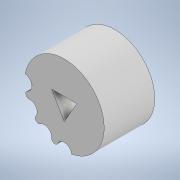
# Autodesk Inventor part: HandleGear
Saved by Autodesk Inventor 2021 (Build 250183000, 183)
## iProperties
Created: 2021-03-14
Part Number: HandleGear
Material: Generic
Document SubType Name: Modeling
Designer: ben
Density: 1 g/cm^3
Appearance: Default
Author: ben
Autodesk Inventor part; units mm, degrees
ref_plane "YZ Plane" through (0, 0, 0) normal (1, 0, 0) x (0, 1, 0)
ref_plane "XZ Plane" through (0, 0, 0) normal (0, 1, 0) x (-1, 0, 0)
ref_plane "XY Plane" through (0, 0, 0) normal (0, 0, 1) x (1, 0, 0)
sketch "Sketch1" plane through (0, 0, 0) normal (0, 0, 1) x (1, 0, 0)
  line L0 (4.323, -2.5122) -> (-0.0282, -10) projected
  line L1 (-0.0282, -10) -> (-4.3372, -2.4878) projected
  line L2 (-8.6461, 5.0244) -> (0.0141, 5) projected
  circle A0 centre (0, 0) radius 27.5 projected
  circle A1 centre (0, 0) radius 22.5
  line L3 (0, 27.5) -> (0, 14.4902)
  line L4 (0, 0) -> (27.5, 0) construction
  line L5 (0, 0) -> (27.5, 0) construction
  circle A2 centre (-27.5, 0) radius 5
  circle A3 centre (-23.8157, -13.75) radius 5
  circle A4 centre (-13.75, -23.8157) radius 5
  circle A5 centre (0, -27.5) radius 5
  line L6 (-4.3372, -2.4878) -> (-8.6461, 5.0244) projected
  line L7 (0.0141, 5) -> (8.6743, 4.9755) projected
  line L8 (8.6743, 4.9755) -> (4.323, -2.5122) projected
  point P0 (0, 0)
  point P1 (-27.0822, 4.7753)
  point P2 (4.7753, -27.0822)
  point P3 (-4.9793, -27.0455)
  point P4 (4.9793, -27.0455)
  point P5 (-27.0455, 4.9793)
  point P6 (-27.0455, -4.9793)
  point P7 (-25.9117, -9.2105)
  point P8 (-20.9324, -17.8349)
  point P9 (-17.8349, -20.9324)
  point P10 (-9.2105, -25.9117)
  point P11 (0, -22.5)
  point P12 (-11.25, -19.4856)
  point P13 (-19.4856, -11.25)
  point P14 (-22.5, 0)
  point P15 (-27.0455, 4.9793)
  point P16 (4.9793, -27.0455)
  dimension "d9" = 10
  dimension "d0" = 5
  dimension "d12" = 90
  constraints: 6 end point, 6 point on circle, 3 centre point, 2 horizontal, 2 vertical, 13 other
  measures "d0" radial gap between concentric circles of A0 A1
extrude "Extrusion1" add sketch "Sketch1" along normal blind 35 contours A0 A5 A1 L3 | L3 A1 A2 A0 | A1 | A0 A4 A1 A5 | A2 A1 A3 A0 | A4 A0 A3 A1
fillet "Fillet6" radius 2 6 edges at (-27.0455, -4.9793, 17.5) (-25.9117, -9.2105, 17.5) (-20.9324, -17.8349, 17.5) (-17.8349, -20.9324, 17.5) (-9.2105, -25.9117, 17.5) (-4.9793, -27.0455, 17.5)
sketch "Sketch5" plane through (0, 0, 35) normal (0, 0, 1) x (1, 0, 0)
  point P0 (0, 0)
body "Solid1"
